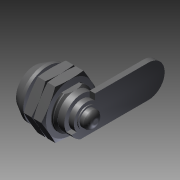
# Autodesk Inventor part: LOCNL2_1
Saved by Autodesk Inventor 2011 SP1 (Build 150282100, 282)
## iProperties
Created: 2015-03-21
Part Number: LOCNL2_1
Catalog Web Link: www.cadenas.de
Description: LOCNL_1-Knuckle Locks
Vendor: MISUMI
Document SubType Name: Modeling
Designer: PARTuser1
Manufacturer: MISUMI
Mass: 2.10859 g
Surface Area: 19.5046 cm^2
Volume: 2.10859 cm^3
Density: 1 g/cm^3
Category: PARTsolutions
Company: MISUMI
Title: LOCNL2_1
Author: Cadenas PARTsolutions
Comments: Knuckle Locks
PSOL_IDENT_0: {\\10.0.0.236\data_v8\23d-libs\misumi\metric\44_handles_hinges\locnl_1.prj},159 {VTYP=3D},{NB=LOCNL2
PSOL_IDENT_1: _1},{LINA=LOCNL2_1},{NN=LOCNL_1},{DATE=14.11.2014 09:15:19},{GEOMDATE=31.03.2009 10:14:00},{VERSION=
PSOL_IDENT_2: },{LINEID=20},{LINESUBID=-1},{WBVAR=}  {NB=LOCNL2_1},{LINA=LOCNL2_1},{KT=DUMMY},{PN=LOCNL2},{TYPE=LO
PSOL_IDENT_3: CNL},{MATMB=Zinc Die Casting},{MATHN=Low Carbon Steel},{MATLP=Low Carbon Steel},{MATK=Low Carbon Ste
PSOL_IDENT_4: el},{STMB=Chrome Plating},{STHN=Trivalent Chromate},{STLP=Trivalent Chromate},{STK=Chrome Plating},{
PSOL_IDENT_5: NO=2},{KD=2  Holes},{MASS=25},{AK=2 Pcs.}
SUPPLIER: MISUMI
ARTICLENO: LOCNL2_1
BOMINFO: LOCNL2_1
CREATOR: CADENAS GmbH
Autodesk Inventor part; units mm, degrees
ref_plane "YZ Plane" through (0, 0, 0) normal (1, 0, 0) x (0, 1, 0)
ref_plane "XZ Plane" through (0, 0, 0) normal (0, 1, 0) x (-1, 0, 0)
ref_plane "XY Plane" through (0, 0, 0) normal (0, 0, 1) x (1, 0, 0)
sketch "Sketch_2" plane through (0, 0, 0) normal (0, 0, 1) x (1, 0, 0)
  line L0 (4, 0) -> (0, 0)
  line L1 (0, 0) -> (0, 5.75)
  line L2 (0, 5.75) -> (3, 7.5)
  line L3 (3, 7.5) -> (4, 7.5)
  line L4 (4, 7.5) -> (4, 0)
  line L5 (4, 0) -> (0, 0)
  constraints: 12 end point
revolve "Revolution1" add sketch "Sketch_2" angle 360 about axis through (4, 0, 0) along (1, 0, 0)
sketch "Sketch_5" plane through (0, 0, 0) normal (0, 0, 1) x (1, 0, 0)
  line L0 (12.5, 0) -> (4, 0)
  line L1 (4, 0) -> (4, 6)
  line L2 (4, 6) -> (11.8865, 6)
  line L3 (11.8865, 6) -> (12.5, 5.3865)
  line L4 (12.5, 5.3865) -> (12.5, 0)
  line L5 (12.5, 0) -> (4, 0)
  constraints: 12 end point
revolve "Revolution2" add sketch "Sketch_5" angle 360 about axis through (12.5, 0, 0) along (1, 0, 0)
thread "Thread1" size "M12x1" class "6g" standard "ISO Metric profile" full length
sketch "Sketch_13" plane through (12.5, 0, 0) normal (1, 0, 0) x (0, 0, -1)
  line L0 (-10, -20) -> (10, -20)
  line L1 (10, -20) -> (10, 20)
  line L2 (10, 20) -> (-10, 20)
  line L3 (-10, 20) -> (-10, -20)
  line L4 (-5.35, -10) -> (5.35, -10)
  line L5 (5.35, -10) -> (5.35, 10)
  line L6 (5.35, 10) -> (-5.35, 10)
  line L7 (-5.35, 10) -> (-5.35, -10)
  constraints: 16 end point
extrude "Extrusion1" cut sketch "Sketch_13" against normal blind 8.5
sketch "Sketch_1" plane through (0, 0, 0) normal (0, 0, 1) x (1, 0, 0)
  line L0 (8, 0) -> (5, 0)
  line L1 (5, 0) -> (5, 7.5)
  line L2 (5, 7.5) -> (5.4019, 9)
  line L3 (5.4019, 9) -> (7.5981, 9)
  line L4 (7.5981, 9) -> (8, 7.5)
  line L5 (8, 7.5) -> (8, 0)
  line L6 (8, 0) -> (5, 0)
  constraints: 14 end point
revolve "Revolution3" add sketch "Sketch_1" angle 360 about axis through (8, 0, 0) along (1, 0, 0)
sketch "Sketch_4" plane through (0, 0, 0) normal (0, 0, 1) x (1, 0, 0)
  line L0 (11, 0) -> (8, 0)
  line L1 (8, 0) -> (8, 7.5)
  line L2 (8, 7.5) -> (8.4019, 9)
  line L3 (8.4019, 9) -> (10.5981, 9)
  line L4 (10.5981, 9) -> (11, 7.5)
  line L5 (11, 7.5) -> (11, 0)
  line L6 (11, 0) -> (8, 0)
  constraints: 14 end point
revolve "Revolution4" add sketch "Sketch_4" angle 360 about axis through (11, 0, 0) along (1, 0, 0)
sketch "Sketch_3" plane through (5, 0, 0) normal (1, 0, 0) x (0, 0, -1)
  line L0 (-15, -15) -> (15, -15)
  line L1 (15, -15) -> (15, 15)
  line L2 (15, 15) -> (-15, 15)
  line L3 (-15, 15) -> (-15, -15)
  line L4 (-7.5, 4.3301) -> (-7.5, -4.3301)
  line L5 (-7.5, -4.3301) -> (0, -8.6603)
  line L6 (0, -8.6603) -> (7.5, -4.3301)
  line L7 (7.5, -4.3301) -> (7.5, 4.3301)
  line L8 (7.5, 4.3301) -> (0, 8.6603)
  line L9 (0, 8.6603) -> (-7.5, 4.3301)
  constraints: 20 end point
extrude "Extrusion2" cut sketch "Sketch_3" along normal blind 6
sketch "Sketch_7" plane through (0, 0, 0) normal (1, 0, 0) x (0, 1, 0)
  circle A0 centre (0, 0) radius 3.707
  constraints: 1 centre point
extrude "Extrusion3" cut sketch "Sketch_7" along normal blind 12.5
sketch "Sketch_6" plane through (0, 0, 0) normal (0, 0, 1) x (1, 0, 0)
  line L0 (14.5, 0) -> (12.5, 0)
  line L1 (12.5, 0) -> (12.5, 5.35)
  line L2 (12.5, 5.35) -> (14.5, 5.35)
  line L3 (14.5, 5.35) -> (14.5, 0)
  line L4 (14.5, 0) -> (12.5, 0)
  constraints: 10 end point
revolve "Revolution5" add sketch "Sketch_6" angle 360 about axis through (14.5, 0, 0) along (1, 0, 0)
sketch "Sketch_8" plane through (0, 0, 0) normal (0, 0, 1) x (1, 0, 0)
  line L0 (14.5, 0) -> (12.5, 0)
  line L1 (12.5, 0) -> (12.5, 1.5)
  line L2 (12.5, 1.5) -> (12.7705, 1.2295)
  line L3 (12.7705, 1.2295) -> (14.2295, 1.2295)
  line L4 (14.2295, 1.2295) -> (14.5, 1.5)
  line L5 (14.5, 1.5) -> (14.5, 0)
  line L6 (14.5, 0) -> (12.5, 0)
  constraints: 14 end point
revolve "Revolution6" cut sketch "Sketch_8" angle 360 about axis through (14.5, 0, 0) along (1, 0, 0)
thread "Thread2" size "M3x0.5" class "6H" standard "ISO Metric profile" full length
sketch "Sketch_9" plane through (0, 0, 0) normal (1, 0, 0) x (0, 1, 0)
  line L0 (0, 0.55) -> (0, -0.55)
  line L1 (0, -0.55) -> (4.6009, -0.55)
  line L2 (4.6009, -0.55) -> (4.6009, 0.55)
  line L3 (4.6009, 0.55) -> (0, 0.55)
  constraints: 8 end point
extrude "Extrusion4" cut sketch "Sketch_9" along normal blind 0.5
sketch "Sketch_10" plane through (0, 0, 0) normal (1, 0, 0) x (0, 1, 0)
  line L0 (0.55, 4.6009) -> (-0.55, 4.6009)
  line L1 (-0.55, 4.6009) -> (-0.55, 0)
  line L2 (-0.55, 0) -> (0.55, 0)
  line L3 (0.55, 0) -> (0.55, 4.6009)
  constraints: 8 end point
extrude "Extrusion5" cut sketch "Sketch_10" along normal blind 0.5
sketch "Sketch_14" plane through (14.5, 0, 0) normal (1, 0, 0) x (0, 0, -1)
  line L0 (-5, 19) -> (-5, 2.5)
  line L1 (-5, 2.5) -> (-3.1225, 2.5)
  arc A0 (-3.1225, 2.5) -> (2.5, -3.1225) centre (0, 0) ccw
  line L2 (2.5, -3.1225) -> (2.5, -4.73)
  arc A1 (2.5, -4.73) -> (5, -1.9033) centre (0, 0) ccw
  line L3 (5, -1.9033) -> (5, 19)
  arc A2 (5, 19) -> (-5, 19) centre (0, 19) ccw
  constraints: 8 end point, 6 point on circle, 3 centre point
extrude "Extrusion6" add sketch "Sketch_14" along normal blind 1.6
sketch "Sketch_15" plane through (0, 0, 0) normal (0, 0, 1) x (1, 0, 0)
  line L0 (18.8, 0) -> (16.1, 0)
  line L1 (16.1, 0) -> (16.1, 3)
  line L2 (16.1, 3) -> (16.4, 3)
  line L3 (16.4, 3) -> (16.4, 2.5)
  line L4 (16.4, 2.5) -> (17.607, 2.5)
  arc A0 (18.8, 0.5) -> (17.607, 2.5) centre (16.692, 0.5984) ccw
  line L5 (18.8, 0.5) -> (18.8, 0)
  line L6 (18.8, 0) -> (16.1, 0)
  constraints: 14 end point, 2 point on circle, 1 centre point
revolve "Revolution7" add sketch "Sketch_15" angle 360 about axis through (18.8, 0, 0) along (1, 0, 0)
ref_plane "1_to_k_XY" through (0.5, 0, 0) normal (1, 0, 0) x (0, 0, -1)
ref_plane "1_to_k_YZ" through (0.5, 0, 0) normal (0, 0, -1) x (0, 1, 0)
ref_plane "1_to_k_ZX" through (0.5, 0, 0) normal (0, 1, 0) x (1, 0, 0)
ref_plane "1_TO_2_XY" through (0, 0, 0) normal (1, 0, 0) x (0, 0, -1)
ref_plane "1_TO_2_YZ" through (0, 0, 0) normal (0, 0, -1) x (0, 1, 0)
ref_plane "1_TO_2_ZX" through (0, 0, 0) normal (0, 1, 0) x (1, 0, 0)
body "Solid1"
